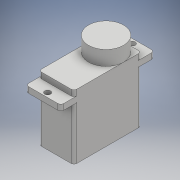
# Autodesk Inventor part: MicroServo
Saved by Autodesk Inventor 2018 (Build 220112000, 112)
## iProperties
Created: 2020-03-23
Part Number: MicroServo
Material: Generic
Document SubType Name: Modeling
Designer: technik
Density: 1 g/cm^3
Appearance: Default
Mass: 6.82204 g
Surface Area: 25.0558 cm^2
Volume: 6.82204 cm^3
Author: technik
Autodesk Inventor part; units mm, degrees
ref_plane "YZ Plane" through (0, 0, 0) normal (1, 0, 0) x (0, 1, 0)
ref_plane "XZ Plane" through (0, 0, 0) normal (0, 1, 0) x (-1, 0, 0)
sketch "Sketch1" plane through (0, 0, 0) normal (0, 0, 1) x (1, 0, 0)
  line L0 (-6, 11.5) -> (6, 11.5)
  line L1 (6, 11.5) -> (6, -11.5)
  line L2 (6, -11.5) -> (-6, -11.5)
  line L3 (-6, -11.5) -> (-6, 11.5)
  line L4 (0, 0) -> (0, -6.2119)
  line L5 (0, 0) -> (2.7529, 0)
  dimension "d0" = 12
  dimension "d1" = 23
  constraints: 12 end point, 2 horizontal, 2 parallel, 1 perpendicular, 2 other
  measures "d0" distance of L0.start L0.end
  measures "d1" distance of L0.end L1.end
extrude "Extrusion1" add sketch "Sketch1" along normal blind 22
ref_plane "Work Plane1" through (0, 0, 20) normal (0, 0, 1) x (1, 0, 0)
sketch "Sketch2" plane through (0, 0, 20) normal (0, 0, 1) x (1, 0, 0)
  line L0 (6, 11.5) -> (-6, 11.5) projected
  line L1 (-6, 11.5) -> (6, 11.5)
  line L2 (6, 11.5) -> (6, 16)
  line L3 (6, 16) -> (-6, 16)
  line L4 (-6, 16) -> (-6, 11.5)
  line L5 (6, -11.5) -> (6, 11.5) projected
  point P0 (0, 0)
  dimension "d5" = 4.5
  constraints: 8 end point, 2 parallel, 1 collinear, 1 horizontal, 1 perpendicular
  measures "d5" distance between parallel lines of L0 L3
extrude "Extrusion2" add sketch "Sketch2" against normal blind 2
sketch "Sketch3" plane through (0, 0, 20) normal (0, 0, 1) x (1, 0, 0)
  circle A0 centre (0, 14.5) radius 1
  line L0 (6, 16) -> (-6, 16) projected
  point P0 (0, 0)
  dimension "d8" = 2
  dimension "d9" = 1.5
  constraints: 1 centre point
  measures "d8" diameter of A0
  measures "d9" distance from line of L0 A0.centre
extrude "Extrusion3" cut sketch "Sketch3" against normal blind 2
fillet "Fillet1" radius 1 6 edges at (6, 16, 19) (-6, 16, 19) (6, 11.5, 9) (6, 11.5, 21) (-6, 11.5, 21) (-6, 11.5, 9)
mirror "Mirror1" about plane through (0, 0, 0) normal (0, 1, 0) of "Extrusion2", "Extrusion3", "Fillet1"
fillet_without_effect "Fillet2"
sketch "Sketch4" plane through (0, 0, 22) normal (0, 0, 1) x (1, 0, 0)
  circle A0 centre (0, 5.5) radius 6
  line L0 (5, 11.5) -> (-5, 11.5) projected
  point P0 (0, 0)
  dimension "d14" = 12
  constraints: 1 centre point, 1 tangent
  measures "d14" diameter of A0
extrude "Extrusion4" add sketch "Sketch4" along normal blind 5
body "Solid1"
